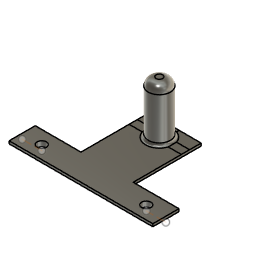
MicroMouse_Balance v6 (Autodesk Fusion 360 design; units mm, degrees)
Autodesk Fusion 360 part; units mm, degrees
sketch "Sketch1" plane through (0, 0, 0) normal (0, 0, 1) x (1, 0, 0)
  line L0 (-27.5, 5) -> (27.5, 5)
  line L1 (27.5, 5) -> (27.5, -5)
  line L2 (27.5, -5) -> (-27.5, -5)
  line L3 (-27.5, -5) -> (-27.5, 5)
  line L4 (-27.5, 5) -> (27.5, -5) construction
  line L5 (27.5, 5) -> (-27.5, -5) construction
  dimension "d1" = 55
  dimension "d2" = 10
  constraint horizontal L0
  constraint perpendicular L0 L1
  constraint parallel L0 L2
  constraint parallel L1 L3
  constraint coincident L4 origin
  constraint coincident L5 origin
  measures "d1" distance of L1.end L2.end
  measures "d2" distance of L0.end L1.end
sketch "Sketch2" plane through (0, 0, 0) normal (0, 0, 1) x (1, 0, 0)
  line L0 (-27.5, 0) -> (-20, 0) construction
  line L1 (27.5, 0) -> (20, 0) construction
  dimension "d3" = 7.5
  dimension "d4" = 7.5
  constraint horizontal L0
  constraint horizontal L1
  measures "d3" distance of L0.start L0.end
  measures "d4" distance of L1.start L1.end
sketch "Sketch3" plane through (0, 0, 0) normal (0, 0, 1) x (1, 0, 0)
  circle A0 centre (-20, 0) radius 1.8
  circle A1 centre (20, 0) radius 1.8
  dimension "d7" = 3.6
  dimension "d8" = 3.6
  measures "d7" diameter of A0
  measures "d8" diameter of A1
extrude "Extrude1" add sketch "Sketch1" along normal blind 2
extrude "Extrude2" cut sketch "Sketch3" along normal blind 10
sketch "Sketch5" plane through (0, 5, 0) normal (0, 1, 0) x (-1, 0, 0)
  line L0 (-27.5, 0) -> (27.5, 0)
  line L1 (27.5, 0) -> (27.5, 2)
  line L2 (27.5, 2) -> (-27.5, 2)
  line L3 (-27.5, 2) -> (-27.5, 0)
  line L4 (-5, 2) -> (5, 2)
  line L5 (5, 2) -> (5, 0)
  line L6 (5, 0) -> (-5, 0)
  line L7 (-5, 0) -> (-5, 2)
  constraint horizontal L4
  constraint vertical L5
  constraint horizontal L6
  constraint vertical L7
  constraint coincident L0 L5.end
  constraint coincident L2 L4.start
extrude "Extrude3" add sketch "Sketch5" along normal blind 25 contours L0 L2 L4 L5 L6 L7
sketch "Sketch6" plane through (0, 0, 2) normal (0, 0, 1) x (-1, 0, 0)
  circle A0 centre (-20, 0) radius 1.8
  circle A1 centre (20, 0) radius 1.8
  line L0 (27.5, 5) -> (-27.5, 5)
  line L1 (-27.5, 5) -> (-27.5, -5)
  line L2 (-27.5, -5) -> (-5, -5)
  line L3 (-5, -5) -> (-5, -30)
  line L4 (-5, -30) -> (5, -30)
  line L5 (5, -30) -> (5, -5)
  line L6 (5, -5) -> (27.5, -5)
  line L7 (27.5, -5) -> (27.5, 5)
  circle A2 centre (0, -25) radius 4.2426
extrude "Extrude4" add sketch "Sketch6" along normal blind 20 contours A2
fillet "Fillet1" radius 3 1 edges at (3.9555, 26.5342, 22)
fillet "Fillet2" radius 1 1 edges at (3.9555, 23.4658, 2)
chamfer "Chamfer1" distance 1 angle 45 8 edges at (-5, 17.5, 0) (5, 17.5, 0) (0, 30, 0) (-16.25, 5, 0) (-27.5, 0, 0) (0, -5, 0) (27.5, 0, 0) (16.25, 5, 0)
extrude "Extrude5" add 1 faces at (-5, 19.4745, 1.3333) along direction (-1, 0, 0) blind 5
extrude "Extrude6" add 1 faces at (5, 19.4745, 1.3333) along direction (1, 0, 0) blind 5
extrude "Extrude7" add 1 faces at (0.5255, 30, 1.3333) along direction (0, 1, 0) blind 5
extrude "Extrude8" cut 1 faces at (1.6667, 35, 1.3333) along direction (0, -1, 0) blind 4
